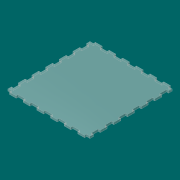
# Autodesk Inventor part: topBottomPanel
Saved by Autodesk Inventor 2016 (Build 200138000, 138)
## iProperties
Created: 2015-10-05
Part Number: topBottomPanel
Material: Polycarbonate, Clear
Document SubType Name: Modeling
Designer: sawai
Density: 1.2 g/cm^3
Appearance: Polycarbonate - Clear
Author: sawai
Autodesk Inventor part; units mm, degrees
ref_plane "YZ Plane" through (0, 0, 0) normal (1, 0, 0) x (0, 1, 0)
ref_plane "XZ Plane" through (0, 0, 0) normal (0, 1, 0) x (-1, 0, 0)
ref_plane "XY Plane" through (0, 0, 0) normal (0, 0, 1) x (1, 0, 0)
sketch "Sketch1" plane through (0, 0, 0) normal (0, 0, 1) x (1, 0, 0)
  line L0 (-60, -60) -> (60, -60)
  line L1 (60, -60) -> (60, 60)
  line L2 (60, 60) -> (-60, 60)
  line L3 (-60, 60) -> (-60, -60)
  line L4 (-60, -60) -> (60, 60) construction
  line L5 (60, -60) -> (-60, 60) construction
  point P0 (0, 0)
  dimension "d0" = 120
  dimension "d1" = 120
  constraints: 12 end point, 2 midpoint, 2 parallel, 1 horizontal, 1 perpendicular
  measures "d0" distance of L2.end L1.end
  measures "d1" distance of L1.end L0.end
extrude "Extrusion1" add sketch "Sketch1" along normal blind 3.175
sketch "Sketch5" plane through (0, 0, 3.175) normal (0, 0, 1) x (1, 0, 0)
  line L0 (-60, -60) -> (60, -60) projected
  line L1 (60, -60) -> (60, 60) projected
  line L2 (60, 60) -> (-60, 60) projected
  line L3 (-60, 60) -> (-60, -60) projected
  line L4 (-60, -60) -> (60, -60) projected
  line L5 (55, -60) -> (45, -60)
  line L6 (45, -60) -> (45, -63.175)
  line L7 (45, -63.175) -> (55, -63.175)
  line L8 (55, -63.175) -> (55, -60)
  point P0 (0, 0)
  dimension "d25" = 10
  dimension "d26" = 3.175
  dimension "d27" = 5
  constraints: 8 end point, 2 parallel, 1 horizontal, 1 perpendicular, 1 point on line
  measures "d25" distance of L6.end L7.end
  measures "d26" distance of L7.end L5.start
  measures "d27" distance between parallel lines of L1 L8
extrude "Extrusion3" add sketch "Sketch5" against normal up to surface (3.175 mm away) contours L0 L8 L7 L6
pattern_linear "Rectangular Pattern2" count 6 spacing 20 along (-1, 0, 0) of "Extrusion3"
mirror "Mirror2" about plane through (0, 0, 0) normal (0, 1, 0) of "Extrusion3", "Rectangular Pattern2"
sketch "Sketch6" plane through (0, 0, 3.175) normal (0, 0, 1) x (1, 0, 0)
  line L0 (-60, -60) -> (-55, -60) projected
  line L1 (-55, -60) -> (-55, -63.175) projected
  line L2 (-55, -63.175) -> (-45, -63.175) projected
  line L3 (-45, -63.175) -> (-45, -60) projected
  line L4 (-45, -60) -> (-35, -60) projected
  line L5 (-35, -60) -> (-35, -63.175) projected
  line L6 (-35, -63.175) -> (-25, -63.175) projected
  line L7 (-25, -63.175) -> (-25, -60) projected
  line L8 (-25, -60) -> (-15, -60) projected
  line L9 (-15, -60) -> (-15, -63.175) projected
  line L10 (-15, -63.175) -> (-5, -63.175) projected
  line L11 (-5, -63.175) -> (-5, -60) projected
  line L12 (-5, -60) -> (5, -60) projected
  line L13 (5, -60) -> (5, -63.175) projected
  line L14 (5, -63.175) -> (15, -63.175) projected
  line L15 (15, -63.175) -> (15, -60) projected
  line L16 (15, -60) -> (25, -60) projected
  line L17 (25, -60) -> (25, -63.175) projected
  line L18 (25, -63.175) -> (35, -63.175) projected
  line L19 (35, -63.175) -> (35, -60) projected
  line L20 (35, -60) -> (45, -60) projected
  line L21 (45, -60) -> (45, -63.175) projected
  line L22 (45, -63.175) -> (55, -63.175) projected
  line L23 (55, -63.175) -> (55, -60) projected
  line L24 (55, -60) -> (60, -60) projected
  line L25 (60, -60) -> (60, 60) projected
  line L26 (60, 60) -> (55, 60) projected
  line L27 (55, 63.175) -> (55, 60) projected
  line L28 (45, 63.175) -> (55, 63.175) projected
  line L29 (45, 60) -> (45, 63.175) projected
  line L30 (45, 60) -> (35, 60) projected
  line L31 (35, 63.175) -> (35, 60) projected
  line L32 (25, 63.175) -> (35, 63.175) projected
  line L33 (25, 60) -> (25, 63.175) projected
  line L34 (25, 60) -> (15, 60) projected
  line L35 (15, 63.175) -> (15, 60) projected
  line L36 (5, 63.175) -> (15, 63.175) projected
  line L37 (5, 60) -> (5, 63.175) projected
  line L38 (5, 60) -> (-5, 60) projected
  line L39 (-5, 63.175) -> (-5, 60) projected
  line L40 (-15, 63.175) -> (-5, 63.175) projected
  line L41 (-15, 60) -> (-15, 63.175) projected
  line L42 (-15, 60) -> (-25, 60) projected
  line L43 (-25, 63.175) -> (-25, 60) projected
  line L44 (-35, 63.175) -> (-25, 63.175) projected
  line L45 (-35, 60) -> (-35, 63.175) projected
  line L46 (-35, 60) -> (-45, 60) projected
  line L47 (-45, 63.175) -> (-45, 60) projected
  line L48 (-55, 63.175) -> (-45, 63.175) projected
  line L49 (-55, 60) -> (-55, 63.175) projected
  line L50 (-55, 60) -> (-60, 60) projected
  line L51 (-60, 60) -> (-60, -60) projected
  line L52 (-60, -55) -> (-56.825, -55)
  line L53 (-56.825, -55) -> (-56.825, -45)
  line L54 (-56.825, -45) -> (-60, -45)
  line L55 (-60, -45) -> (-60, -55)
  point P0 (0, 0)
  dimension "d33" = 3.175
  dimension "d34" = 10
  dimension "d35" = 5
  constraints: 8 end point, 2 parallel, 1 horizontal, 1 perpendicular, 1 point on line
  measures "d33" distance of L53.end L54.end
  measures "d34" distance of L52.end L53.end
  measures "d35" distance between parallel lines of L0 L52
extrude "Extrusion4" cut sketch "Sketch6" against normal up to surface (3.175 mm away) contours L51 L54 L53 L52
pattern_linear "Rectangular Pattern3" count 6 spacing 20 along (0, 1, 0) of "Extrusion4"
mirror "Mirror3" about plane through (0, 0, 0) normal (1, 0, 0) of "Extrusion4", "Rectangular Pattern3"
equation "\"d0\" = width"
equation "\"d1\" = depth"
equation "\"d2\" = materialThickness"
equation "\"d25\" = notchWidth"
equation "\"d26\" = materialThickness"
equation "\"d27\" = 0.5 * notchWidth"
equation "\"d32\" = 2 * notchWidth"
equation "\"d33\" = materialThickness"
equation "\"d34\" = notchWidth"
equation "\"d35\" = 0.5 * notchWidth"
equation "\"d40\" = 2 * notchWidth"
equation "\"width\" = 120"
equation "\"depth\" = 120"
equation "\"materialThickness\" = 3.175"
equation "\"laserKerf\" = 0.1"
equation "\"spoolDiameter\" = 95"
equation "\"cardPinDiameter\" = 3"
equation "\"cardFillet\" = 2.88"
equation "\"cardSelected\" = 1"
equation "\"cardThickness\" = 0.76"
equation "\"cardHeight\" = 53.98"
equation "\"cardWidth\" = 85.6"
equation "\"centeralShaftDiameter\" = 8"
equation "\"cardClearence\" = 0.5"
equation "\"bearingOd\" = 22"
equation "\"bearingWidth\" = 8"
equation "\"axleHeight\" = 95"
equation "\"nutTrapDepth\" = 2.5"
equation "\"nutTrapwidth\" = 5.5"
equation "\"nutTrapClearence\" = 2"
equation "\"magnetLength\" = 3"
equation "\"magnetDiameter\" = 6"
equation "\"magnetProtusion\" = 0.25"
equation "\"notchWidth\" = 10"
equation "\"spoolThickness\" = 5.588"
body "Solid1"
